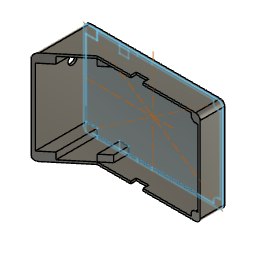
Assignment (Autodesk Fusion 360 design; units mm, degrees)
Autodesk Fusion 360 part; units mm, degrees
sketch "Sketch1" plane through (0, 0, 0) normal (0, 1, 0) x (1, 0, 0)
  line L0 (0, -6) -> (0, -74)
  line L1 (6, 0) -> (114, 0)
  line L2 (10, -80) -> (114, -80)
  line L3 (120, -74) -> (120, -6)
  line L4 (114, -80) -> (114, -78)
  line L5 (118, -74) -> (120, -74)
  arc A0 (118, -74) -> (114, -78) centre (118, -78) ccw
  line L6 (60, -90) -> (60, 5.1321) construction
  line L7 (0, -40) -> (77.2203, -40) construction
  arc A1 (114, -2) -> (118, -6) centre (118, -2) ccw
  line L8 (118, -6) -> (120, -6)
  line L9 (114, 0) -> (114, -2)
  line L10 (30, -80) -> (30, -74)
  line L11 (30, -74) -> (38, -74)
  line L12 (38, -74) -> (38, -80)
  line L13 (6, -74) -> (0, -74)
  line L14 (30, -80) -> (30, -82)
  line L15 (46, -80) -> (46, -82)
  line L16 (59, -80) -> (59, -82)
  line L17 (0, -74) -> (0, -6)
  line L18 (6, 0) -> (114, 0)
  line L19 (30, 0) -> (30, -6)
  line L20 (30, -6) -> (38, -6)
  line L21 (46, 0) -> (46, 2)
  line L22 (30, 0) -> (30, 2)
  line L23 (38, -6) -> (38, 0)
  line L24 (59, 0) -> (59, 2)
  line L25 (118, -82) -> (2, -82)
  line L26 (-2, -78) -> (-2, -2)
  line L27 (2, 2) -> (118, 2)
  line L28 (122, -2) -> (122, -78)
  line L29 (122, -82) -> (-2, 2) construction
  line L30 (-2, -82) -> (122, 2) construction
  arc A2 (118, -82) -> (122, -78) centre (118, -78) ccw
  arc A3 (-2, -78) -> (2, -82) centre (2, -78) ccw
  arc A4 (2, 2) -> (-2, -2) centre (2, -2) ccw
  arc A5 (122, -2) -> (118, 2) centre (118, -2) ccw
  line L31 (10, -74) -> (10, -80)
  arc A6 (6, -74) -> (9.9896, -74) centre (11.9235, 32231376.4081) ccw
  line L32 (6, -6) -> (0, -6)
  arc A7 (10, -6) -> (6.0104, -6) centre (11.9235, -32231456.4081) ccw
  line L33 (10, -6) -> (10, 0)
  line L34 (10, -80) -> (10, -82)
  line L35 (10, 0) -> (10, 2)
  line L36 (0, -74) -> (0, -81.4641)
  line L37 (10, -74) -> (10, -82)
  arc A8 (0, -6) -> (0, 1.4614) centre (-20307053.8707, -6) ccw
  line L38 (10, -6) -> (0, -6)
  line L39 (0, -19) -> (0, -74)
  line L40 (10, -74) -> (10, -82)
  line L41 (0, -74) -> (10, -74)
  line L42 (10, -82) -> (14, -82)
  line L43 (30, -80) -> (38, -80)
  point P0 (60, -40)
  dimension "d6" = 4
  dimension "d7" = 30
  dimension "d11" = 16
  dimension "d12" = 13
  dimension "d13" = 124
  dimension "d14" = 84
  dimension "d15" = 4
  dimension "d16" = 4
  dimension "d17" = 4
  dimension "d18" = 4
  dimension "d19" = 10
  constraint vertical L0
  constraint perpendicular L0 L1
  constraint perpendicular L0 L2
  constraint vertical L4
  constraint horizontal L5
  constraint tangent L4 A0
  constraint tangent L5 A0
  constraint perpendicular L1 L6
  constraint symmetric L3.start L6 L0.end
  constraint perpendicular L0 L7
  constraint symmetric L2.end L7 L1.end
  constraint symmetric L3.start L7 L3.end
  constraint symmetric L4.end L7 A1.start
  constraint symmetric L5.start L7 A1.end
  constraint symmetric A0 L7 A1
  constraint symmetric L0.end L7 L0.start
  constraint coincident L0 L7.start
  constraint coincident L2 L10.start
  constraint perpendicular L2 L10
  constraint perpendicular L10 L11
  constraint perpendicular L11 L12
  constraint perpendicular L2 L14
  constraint coincident L2 L15.start
  constraint perpendicular L2 L15
  constraint coincident L2 L16.start
  constraint perpendicular L2 L16
  constraint symmetric L7 L0.start L0.end
  constraint symmetric L7 L10.start L19.start
  constraint symmetric L7 L10.end L19.end
  constraint symmetric L7 L11.end L20.end
  constraint symmetric L7 L12.end L23.end
  constraint symmetric L7 L14.end L22.end
  constraint symmetric L7 L15.start L21.start
  constraint symmetric L7 L15.end L21.end
  constraint symmetric L7 L16.start L24.start
  constraint symmetric L7 L16.end L24.end
  constraint horizontal L25
  constraint perpendicular L25 L26
  constraint parallel L25 L27
  constraint parallel L26 L28
  constraint coincident L29 P0
  constraint coincident L30 P0
  constraint coincident L7 P0
  constraint coincident L6 P0
  constraint coincident L29.start L25
  constraint coincident L29.start L28
  constraint tangent L25 A2
  constraint tangent L28 A2
  constraint coincident L30.start L26
  constraint coincident L30.start L25
  constraint tangent L26 A3
  constraint tangent L25 A3
  constraint coincident L29.end L26
  constraint coincident L29.end L27
  constraint tangent L26 A4
  constraint tangent L27 A4
  constraint coincident L30.end L27
  constraint coincident L30.end L28
  constraint tangent L27 A5
  constraint tangent L28 A5
  constraint perpendicular L2 L31
  constraint tangent L13 A6
  constraint symmetric L7 L13.start L32.start
  constraint symmetric L7 L31.start A7.start
  constraint symmetric L7 L2.start L33.end
  constraint symmetric L7 A6 A7
  constraint coincident L25 L34.end
  constraint perpendicular L25 L34
  constraint coincident L27 L35.end
  constraint perpendicular L27 L35
  constraint coincident A3 L36.end
  constraint perpendicular L25 L36
  constraint tangent L0 A8
  constraint coincident L0 L39.start
  constraint coincident L25 L42.end
  constraint perpendicular L10 L43
  measures "d6" radius of A0
  measures "d7" distance of L0 L10
  measures "d11" distance of L14 L15
  measures "d12" distance of L15 L16
  measures "d13" distance of L29.end L30.end
  measures "d14" distance of L30.start L29.end
  measures "d15" radius of A2
  measures "d16" radius of A3
  measures "d17" radius of A4
  measures "d18" radius of A5
  measures "d19" distance of L17 L31
extrude "Extrude1" add sketch "Sketch1" along normal blind 2 makes body 1
extrude "Extrude3" add sketch "Sketch1" against normal blind 20 contours L1 L18 L19 L20 L23 bodies 1
extrude "Extrude4" add sketch "Sketch1" against normal blind 20 contours L0 L17 L26 L27 A3 A4 L32 A7 L33 L35 L36 L38 L39 | L13 L25 A3 L31 A6 L34 L36 L37 L40 L41 | L1 L18 L22 L27 L35 | L2 L14 L25 L34 L37 L40 L42 | L1 L18 L21 L22 L27 | L2 L10 L11 L12 L43 | L2 L14 L15 L25 L43 bodies 1
extrude "Extrude5" add sketch "Sketch1" against normal blind 20 contours L1 L18 L21 L24 L27 | L2 L15 L16 L25 | L1 L2 L3 L4 L5 A0 A1 L8 L9 L16 L18 L24 L25 L27 L28 A2 A5 bodies 1
sketch "Sketch3" plane through (0, -20, 0) normal (0, -1, 0) x (1, 0, 0)
  line L0 (114, 0) -> (38, 0)
  line L1 (38, 0) -> (38, 6)
  line L2 (38, 6) -> (30, 6)
  line L3 (30, 6) -> (30, 0)
  line L4 (30, 0) -> (10, 0)
  line L5 (10, 0) -> (10, 6)
  line L6 (10, 6) -> (0, 6)
  line L7 (0, 6) -> (0, 74)
  line L8 (0, 74) -> (10, 74)
  line L9 (10, 74) -> (10, 80)
  line L10 (10, 80) -> (30, 80)
  line L11 (30, 80) -> (30, 74)
  line L12 (30, 74) -> (38, 74)
  line L13 (38, 74) -> (38, 80)
  line L14 (38, 80) -> (114, 80)
  line L15 (114, 80) -> (114, 78)
  arc A0 (114, 78) -> (118, 74) centre (118, 78) ccw
  line L16 (118, 74) -> (120, 74)
  line L17 (120, 74) -> (120, 6)
  line L18 (120, 6) -> (118, 6)
  arc A1 (118, 6) -> (114, 2) centre (118, 2) ccw
  line L19 (114, 2) -> (114, 0)
  line L20 (2, -2) -> (118, -2)
  arc A2 (118, -2) -> (122, 2) centre (118, 2) ccw
  line L21 (122, 2) -> (122, 78)
  arc A3 (122, 78) -> (118, 82) centre (118, 78) ccw
  line L22 (118, 82) -> (2, 82)
  arc A4 (2, 82) -> (-2, 78) centre (2, 78) ccw
  line L23 (-2, 78) -> (-2, 2)
  arc A5 (-2, 2) -> (2, -2) centre (2, 2) ccw
  line L24 (30, 0) -> (30, -2)
  line L25 (30, 82) -> (30, 80)
  line L26 (30, 80) -> (10, 80)
  line L27 (10, 74) -> (0, 74)
  line L28 (0, 6) -> (10, 6)
  constraint coincident L3.end L4.start
  constraint coincident L20 L24.end
  constraint perpendicular L20 L24
  constraint coincident L22 L25.start
  constraint perpendicular L22 L25
  constraint coincident L10.end L11.start
  constraint coincident L9.end L10.start
  constraint coincident L8.end L9.start
  constraint coincident L7.end L8.start
  constraint coincident L6.end L7.start
  constraint coincident L5.end L6.start
extrude "Extrude6" add sketch "Sketch3" along normal blind 30 contours L4 L5 L6 L7 L8 L9 L10 L20 L22 A4 L23 A5 L24 L25 L26 L27 L28 bodies 1
sketch "Sketch4" plane through (0, 0, -2) normal (0, 0, -1) x (1, 0, 0)
  line L0 (2, 50) -> (2, -2)
  line L1 (2, -2) -> (118, -2)
  line L2 (118, -2) -> (118, 20)
  line L3 (118, 20) -> (30, 20)
  line L4 (30, 20) -> (30, 50)
  line L5 (30, 50) -> (2, 50)
  line L6 (30, 20) -> (-46.6044, 84.2788)
  line L7 (30, 20) -> (31, 20) construction
  dimension "d32" = 140
  dimension "d33" = 100
  constraint horizontal L7
  constraint coincident L3.end L4.start
  measures "d32" angle of L6 L7
  measures "d33" distance of L3.end L6.end
extrude "Extrude7" cut sketch "Sketch4" against normal blind 100 contours L0 L4 L5 L6 bodies 1
extrude "Extrude8" cut 1 faces at (-1.3333, -50, 51.3333) along direction (0, -1, 0) up to surface end surface through (10, -36.782, 3) normal (0.642788, -0.766044, 0) offset 0 on bodies 1 bodies 1
sketch "Sketch6" plane through (0, 0, -2) normal (0, 0, -1) x (1, 0, 0)
  line L0 (60, 20) -> (60, 15)
  line L1 (60, 15) -> (71, 15)
  line L2 (71, 15) -> (71, 20)
  line L3 (71, 20) -> (60, 20)
  point P0 (30, 20)
  dimension "d39" = 11
  dimension "d40" = 30
  constraint vertical L0
  constraint perpendicular L0 L1
  constraint perpendicular L1 L2
  constraint perpendicular L0 L3
  measures "d39" distance of L0.end L1.end
  measures "d40" distance of L0 P0
extrude "Extrude9" cut sketch "Sketch6" against normal blind 120 bodies 1
sketch "Sketch8" plane through (0, -20, 0) normal (0, -1, 0) x (1, 0, 0)
  line L0 (60, 80) -> (60, 82)
  line L1 (60, 82) -> (30, 82)
  line L2 (30, 82) -> (30, 80)
  line L3 (30, 80) -> (30, 74)
  line L4 (30, 74) -> (38, 74)
  line L5 (38, 74) -> (38, 80)
  line L6 (38, 80) -> (60, 80)
  line L7 (38, 80) -> (30, 80)
  constraint coincident L5.end L6.start
  constraint coincident L2.end L3.start
extrude "Extrude10" cut sketch "Sketch8" against normal blind 13 contours L3 L4 L5 L7 bodies 1
extrude "Extrude11" add 1 faces at (32.6667, -7, 76) along direction (0, -1, 0) up to surface end surface through (30, -20, 77) normal (0.642788, -0.766044, 0) offset 0 on bodies 1 bodies 1
sketch "Sketch10" plane through (0, -20, 0) normal (0, -1, 0) x (1, 0, 0)
  line L0 (60, -2) -> (60, 0)
  line L1 (60, 0) -> (38, 0)
  line L2 (38, 0) -> (38, 6)
  line L3 (38, 6) -> (30, 6)
  line L4 (30, 6) -> (30, 0)
  line L5 (30, 0) -> (30, -2)
  line L6 (30, -2) -> (60, -2)
  line L7 (38, 0) -> (30, 0)
  constraint coincident L1.end L2.start
  constraint coincident L4.end L5.start
extrude "Extrude12" cut sketch "Sketch10" against normal blind 6 contours L2 L3 L4 L7 bodies 1
extrude "Extrude13" cut 1 faces at (32.6667, -14, 2) along direction (0, 1, 0) blind 3 on bodies 1 bodies 1
extrude "Extrude14" add 1 faces at (32.6667, -11, 2) along direction (0, -1, 0) blind 15 on bodies 1 bodies 1
extrude "Extrude15" add 1 faces at (32.6667, -11.0957, 74) along direction (0, 0, -1) blind 30 from surface at 68 on bodies 1 bodies 1
extrude "Extrude16" cut 1 faces at (35.3333, -8.6667, 6) along direction (0, 0, -1) blind 10 on bodies 1 bodies 1 makes body 2 at (30, -6.6667, -10.6667)
extrude "Extrude17" add 1 faces at (32.6667, -11.0957, -24) along direction (0, 0, 1) blind 30 on bodies 2 bodies 2 1
extrude "Extrude18" cut 1 faces at (32.6667, -11.0957, -24) along direction (0, 0, 1) blind 22 on bodies 2 bodies 2
extrude "Extrude19" add 1 faces at (99.6667, -11.6667, 80) along direction (0, 0, -1) blind 2 from surface at 80 on bodies 2 bodies 2
sketch "Sketch11" plane through (-2, 0, 0) normal (-1, 0, 0) x (0, -1, 0)
  line L0 (46.8512, 2) -> (46.8512, 78)
  line L1 (46.8512, 78) -> (-2, 78)
  line L2 (-2, 78) -> (-2, 2)
  line L3 (-2, 2) -> (46.8512, 2)
  circle A0 centre (12, 60) radius 4
  dimension "d67" = 8
  dimension "d68" = 18
  dimension "d69" = 14
  measures "d67" diameter of A0
  measures "d68" distance of L1 A0.centre
  measures "d69" distance of L2 A0.centre
extrude "Extrude20" cut sketch "Sketch11" against normal blind 10 contours A0 bodies 2
extrude "Extrude2" [suppressed]
